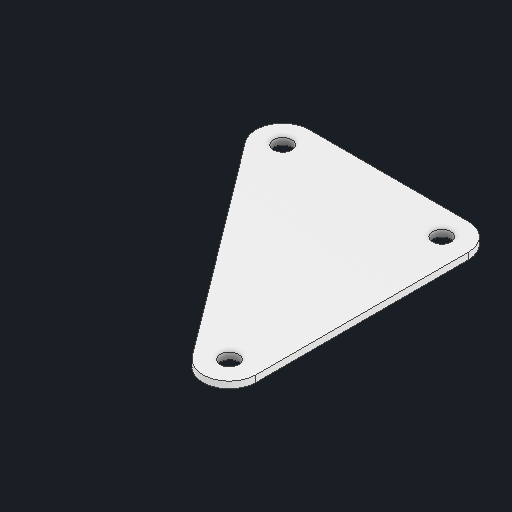
# Autodesk Inventor part: intake_gusset
Saved by Autodesk Inventor 2025 (Build 290162000, 162)
## iProperties
Created: 2024-07-02
Part Number: intake_gusset
Material: Acetal Resin, White
Document SubType Name: Sheet Metal
Designer: Averey Ku
Density: 1.425 g/cm^3
Appearance: Smooth - White
Flat Pattern Width: 4.318 cm
Flat Pattern Length: 7.62 cm
Flat Pattern Area: 32.9032 cm^2
Sheet Metal Rule: Default_mm
Sheet Metal Width: 1.700 in
Sheet Metal Length: 3.000 in
Sheet Metal Area: 5.100 in^2
Author: Averey Ku
Autodesk Inventor part; units mm, degrees
ref_plane "YZ Plane" through (0, 0, 0) normal (1, 0, 0) x (0, 1, 0)
ref_plane "XZ Plane" through (0, 0, 0) normal (0, 1, 0) x (-1, 0, 0)
ref_plane "XY Plane" through (0, 0, 0) normal (0, 0, 1) x (1, 0, 0)
sketch "main" plane through (0, 0, 0) normal (0, 0, 1) x (1, 0, 0)
  circle A0 centre (-17.594, -20.0255) radius 2.1844
  circle A1 centre (20.506, -20.0255) radius 2.1844
  circle A2 centre (-17.594, 30.7745) radius 2.1844
  arc A3 (-23.944, -20.0255) -> (-17.594, -26.3755) centre (-17.594, -20.0255) ccw
  arc A4 (20.506, -26.3755) -> (25.586, -16.2155) centre (20.506, -20.0255) ccw
  arc A5 (-12.514, 34.5845) -> (-23.944, 30.7745) centre (-17.594, 30.7745) ccw
  line L0 (-17.594, -26.3755) -> (20.506, -26.3755)
  line L1 (-23.944, -20.0255) -> (-23.944, 30.7745)
  line L2 (25.586, -16.2155) -> (-12.514, 34.5845)
  point P0 (-7.053, -5.2935)
  dimension "d0" = 12.7
  dimension "d1" = 12.7
  dimension "d2" = 12.7
  measures "d0" diameter of A3
  measures "d1" diameter of A4
  measures "d2" diameter of A5
sketch "Sketch1" plane through (0, 0, 0) normal (0, 1, 0) x (-1, 0, 0)
  circle A0 centre (0, 0) radius 2.1844
  circle A1 centre (38.1, 0) radius 2.1844
  circle A2 centre (0, 50.8) radius 2.1844
  arc A3 (-6.35, 0) -> (0, -6.35) centre (0, 0) ccw
  arc A4 (38.1, -6.35) -> (43.18, 3.81) centre (38.1, 0) ccw
  arc A5 (5.08, 54.61) -> (-6.35, 50.8) centre (0, 50.8) ccw
  line L0 (0, -6.35) -> (38.1, -6.35)
  line L1 (-6.35, 0) -> (-6.35, 50.8)
  line L2 (43.18, 3.81) -> (5.08, 54.61)
  constraints: 1 other
extrude "Extrusion1" add sketch "Sketch1" along normal blind 1.5875
equation "\"BendRadius\" = Thickness"
equation "\"BendReliefWidth\" = Thickness"
equation "\"BendReliefDepth\" = 0.5 * Thickness"
equation "\"CornerReliefSize\" = 4 * Thickness"
equation "\"MinimumRemnant\" = 2 * Thickness"
equation "\"TransitionRadius\" = BendRadius"
equation "\"JacobiRadiusSize\" = BendRadius"
equation "\"GapSize\" = Thickness"
equation "\"Thickness\" = 1.5875"
body "Solid1"
